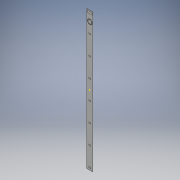
# Autodesk Inventor part: Pieza1
Saved by Autodesk Inventor 2018 (Build 220112000, 112)
## iProperties
Created: 2018-02-27
Part Number: Pieza1
Material: Genérico
Document SubType Name: Modeling
Designer: ivanb
Density: 1 g/cm^3
Appearance: Valor por defecto
Author: ivanb
Autodesk Inventor part; units mm, degrees
ref_plane "YZ Plane" through (0, 0, 0) normal (1, 0, 0) x (0, 1, 0)
ref_plane "XZ Plane" through (0, 0, 0) normal (0, 1, 0) x (-1, 0, 0)
ref_plane "XY Plane" through (0, 0, 0) normal (0, 0, 1) x (1, 0, 0)
sketch "Boceto1" plane through (0, 0, 0) normal (0, 1, 0) x (-1, 0, 0)
  line L0 (-6.5, -143.75) -> (6.5, -143.75)
  line L1 (6.5, -143.75) -> (6.5, 143.75)
  line L2 (6.5, 143.75) -> (-6.5, 143.75)
  line L3 (-6.5, 143.75) -> (-6.5, -143.75)
  line L4 (0, 0) -> (-31.3915, 0)
  line L5 (0, 0) -> (0, -12.323)
  dimension "d0" = 13
  dimension "d1" = 287.5
  constraints: 12 end point, 2 horizontal, 2 parallel, 1 perpendicular, 1 vertical, 2 other
  measures "d0" distance of L2.end L1.end
  measures "d1" distance of L1.end L0.end
extrude "Extrusión1" add sketch "Boceto1" along normal blind 0.16
sketch "Boceto2" plane through (0, 0.16, 0) normal (0, 1, 0) x (1, 0, 0)
  point P0 (0, 0)
sketch "Boceto3" plane through (0, 0.16, 0) normal (0, 1, 0) x (1, 0, 0)
  line L0 (6.5, 143.75) -> (-6.5, 143.75) projected
  line L1 (0, 143.75) -> (0, 97.75)
  line L2 (-2.25, 97.75) -> (2.25, 97.75)
  line L3 (2.25, 97.75) -> (2.25, 100.1)
  line L4 (2.25, 100.1) -> (-2.25, 100.1)
  line L5 (-2.25, 100.1) -> (-2.25, 97.75)
  line L6 (2.25, 57.75) -> (-2.25, 57.75)
  line L7 (-2.25, 57.75) -> (-2.25, 60.1)
  line L8 (-2.25, 60.1) -> (2.25, 60.1)
  line L9 (2.25, 60.1) -> (2.25, 57.75)
  line L10 (2.25, 57.75) -> (-2.25, 60.1) construction
  line L11 (-2.25, 57.75) -> (2.25, 60.1) construction
  line L12 (0, 38.925) -> (-3.2759, 38.925)
  line L13 (0, 78.925) -> (-4.0754, 78.925)
  line L14 (2.25, 20.1) -> (-2.25, 20.1)
  line L15 (-2.25, 20.1) -> (-2.25, 17.75)
  line L16 (-2.25, 17.75) -> (2.25, 17.75)
  line L17 (2.25, 17.75) -> (2.25, 20.1)
  line L18 (2.25, 20.1) -> (-2.25, 17.75) construction
  line L19 (-2.25, 20.1) -> (2.25, 17.75) construction
  line L20 (0, -1.075) -> (-4.0754, -1.075)
  line L21 (0, -41.075) -> (-3.2759, -41.075)
  line L22 (-2.25, -19.9) -> (2.25, -19.9)
  line L23 (2.25, -22.25) -> (-2.25, -22.25)
  line L24 (-2.25, -22.25) -> (-2.25, -19.9)
  line L25 (2.25, -19.9) -> (2.25, -22.25)
  line L26 (-2.25, -22.25) -> (2.25, -19.9) construction
  line L27 (2.25, -22.25) -> (-2.25, -19.9) construction
  line L28 (0, -81.075) -> (-4.0754, -81.075)
  line L29 (2.25, -59.9) -> (-2.25, -59.9)
  line L30 (-2.25, -62.25) -> (2.25, -62.25)
  line L31 (2.25, -62.25) -> (2.25, -59.9)
  line L32 (-2.25, -59.9) -> (2.25, -62.25) construction
  line L33 (2.25, -59.9) -> (-2.25, -62.25) construction
  line L34 (-2.25, -59.9) -> (-2.25, -62.25)
  line L35 (0, -121.075) -> (-3.2759, -121.075)
  line L36 (-2.25, -99.9) -> (2.25, -99.9)
  line L37 (2.25, -102.25) -> (-2.25, -102.25)
  line L38 (2.25, -99.9) -> (2.25, -102.25)
  line L39 (-2.25, -102.25) -> (2.25, -99.9) construction
  line L40 (2.25, -102.25) -> (-2.25, -99.9) construction
  line L41 (-2.25, -102.25) -> (-2.25, -99.9)
  line L42 (0, 118.925) -> (-3.2759, 118.925)
  line L43 (-2.25, 140.1) -> (2.25, 140.1)
  line L44 (2.25, 140.1) -> (2.25, 137.75)
  line L45 (2.25, 137.75) -> (-2.25, 137.75)
  line L46 (-2.25, 137.75) -> (-2.25, 140.1)
  point P0 (0, 0)
  point P1 (0, 98.925)
  point P2 (0, 58.925)
  point P3 (0, 18.925)
  point P4 (0, -21.075)
  point P5 (0, -82.15)
  point P6 (0, -61.075)
  point P7 (0, -101.075)
  point P8 (0, 140.1)
  point P9 (0, 138.925)
  dimension "d4" = 46
  dimension "d5" = 4.5
  dimension "d6" = 2.35
  dimension "d7" = 40
  dimension "d8" = 4.5
  dimension "d9" = 2.35
  dimension "d10" = 20
  dimension "d11" = 20
  constraints: 92 end point, 37 symmetric about line, 11 midpoint, 4 horizontal, 4 parallel, 2 perpendicular, 1 point on line, 1 vertical, 1 other
  measures "d4" distance of L1.start L1.end
  measures "d5" distance of L4.end L3.end
  measures "d6" distance of L3.end L2.end
  measures "d7" distance of point (0, 98.925) point (0, 58.925)
  measures "d8" distance of L6.start L6.end
  measures "d9" distance of L6.end L7.end
  measures "d10" distance from line of L12 point (0, 58.925)
  measures "d11" distance from line of L13 point (0, 98.925)
extrude "Extrusión2" add sketch "Boceto3" along normal blind 1
sketch "Boceto4" plane through (0, 0.16, 0) normal (0, 1, 0) x (1, 0, 0)
  line L0 (-6.5, -143.75) -> (6.5, -143.75) projected
  line L1 (-3.5, -126.25) -> (3.5, -126.25)
  line L2 (3.5, -126.25) -> (3.5, -119.25)
  line L3 (3.5, -119.25) -> (-3.5, -119.25)
  line L4 (-3.5, -119.25) -> (-3.5, -126.25)
  line L5 (-3.5, -126.25) -> (3.5, -119.25) construction
  line L6 (3.5, -126.25) -> (-3.5, -119.25) construction
  point P0 (0, 0)
  point P1 (0, -122.75)
  dimension "d14" = 21
  dimension "d15" = 7
  dimension "d16" = 7
  constraints: 12 end point, 2 midpoint, 2 parallel, 1 horizontal, 1 perpendicular
  measures "d14" distance from line of point (0, -122.75) L0
  measures "d15" distance of L3.end L2.end
  measures "d16" distance of L2.end L1.end
extrude "Extrusión3" add sketch "Boceto4" along normal blind 1
sketch "Boceto5" plane through (0, 0.16, 0) normal (0, 1, 0) x (1, 0, 0)
  line L0 (3.5, -119.25) -> (-3.5, -119.25) projected
  line L1 (-2.7, -119.25) -> (-2.2, -119.25)
  line L2 (-2.2, -119.25) -> (-2.2, -117.9762)
  line L3 (-2.2, -117.9762) -> (-2.7, -117.9762)
  line L4 (-2.7, -117.9762) -> (-2.7, -119.25)
  line L5 (-2, -119.25) -> (-1.5, -119.25)
  line L6 (-1.5, -119.25) -> (-1.5, -117.9762)
  line L7 (-1.5, -117.9762) -> (-2, -117.9762)
  line L8 (-2, -117.9762) -> (-2, -119.25)
  line L9 (-1.3, -119.25) -> (-0.8, -119.25)
  line L10 (-0.8, -119.25) -> (-0.8, -117.9762)
  line L11 (-0.8, -117.9762) -> (-1.3, -117.9762)
  line L12 (-1.3, -117.9762) -> (-1.3, -119.25)
  line L13 (-0.6, -119.25) -> (-0.1, -119.25)
  line L14 (-0.1, -119.25) -> (-0.1, -117.9762)
  line L15 (-0.1, -117.9762) -> (-0.6, -117.9762)
  line L16 (-0.6, -117.9762) -> (-0.6, -119.25)
  line L17 (0.1, -119.25) -> (0.6, -119.25)
  line L18 (0.6, -119.25) -> (0.6, -117.9762)
  line L19 (0.6, -117.9762) -> (0.1, -117.9762)
  line L20 (0.1, -117.9762) -> (0.1, -119.25)
  line L21 (0.8, -119.25) -> (1.3, -119.25)
  line L22 (1.3, -119.25) -> (1.3, -117.9762)
  line L23 (1.3, -117.9762) -> (0.8, -117.9762)
  line L24 (0.8, -117.9762) -> (0.8, -119.25)
  line L25 (1.5, -119.25) -> (2, -119.25)
  line L26 (2, -119.25) -> (2, -117.9762)
  line L27 (2, -117.9762) -> (1.5, -117.9762)
  line L28 (1.5, -117.9762) -> (1.5, -119.25)
  line L29 (2.2, -119.25) -> (2.7, -119.25)
  line L30 (2.7, -119.25) -> (2.7, -117.9762)
  line L31 (2.7, -117.9762) -> (2.2, -117.9762)
  line L32 (2.2, -117.9762) -> (2.2, -119.25)
  line L33 (2.25, -102.25) -> (-2.25, -102.25) projected
  line L34 (0, -102.25) -> (0, -103.6026)
  line L35 (-3.5, -119.25) -> (-3.5, -119.452)
  line L36 (-3.5, -126.25) -> (-3.5, -119.25) projected
  line L37 (-3.5, -119.25) -> (3.5, -119.25) projected
  line L38 (-3.5, -119.25) -> (-3.2852, -119.25)
  line L39 (-3.5, -119.25) -> (-3.5, -126.25) projected
  line L40 (-3.5, -122.75) -> (-4.815, -122.75)
  line L41 (-2.7, -126.25) -> (-2.2, -126.25)
  line L42 (-2.2, -126.25) -> (-2.2, -127.5238)
  line L43 (-2.2, -127.5238) -> (-2.7, -127.5238)
  line L44 (-2.7, -127.5238) -> (-2.7, -126.25)
  line L45 (-2, -126.25) -> (-1.5, -126.25)
  line L46 (-1.5, -126.25) -> (-1.5, -127.5238)
  line L47 (-1.5, -127.5238) -> (-2, -127.5238)
  line L48 (-2, -127.5238) -> (-2, -126.25)
  line L49 (-1.3, -126.25) -> (-0.8, -126.25)
  line L50 (-0.8, -126.25) -> (-0.8, -127.5238)
  line L51 (-0.8, -127.5238) -> (-1.3, -127.5238)
  line L52 (-1.3, -127.5238) -> (-1.3, -126.25)
  line L53 (-0.6, -126.25) -> (-0.1, -126.25)
  line L54 (-0.1, -126.25) -> (-0.1, -127.5238)
  line L55 (-0.1, -127.5238) -> (-0.6, -127.5238)
  line L56 (-0.6, -127.5238) -> (-0.6, -126.25)
  line L57 (0.1, -126.25) -> (0.6, -126.25)
  line L58 (0.6, -126.25) -> (0.6, -127.5238)
  line L59 (0.6, -127.5238) -> (0.1, -127.5238)
  line L60 (0.1, -127.5238) -> (0.1, -126.25)
  line L61 (0.8, -126.25) -> (1.3, -126.25)
  line L62 (1.3, -126.25) -> (1.3, -127.5238)
  line L63 (1.3, -127.5238) -> (0.8, -127.5238)
  line L64 (0.8, -127.5238) -> (0.8, -126.25)
  line L65 (1.5, -126.25) -> (2, -126.25)
  line L66 (2, -126.25) -> (2, -127.5238)
  line L67 (2, -127.5238) -> (1.5, -127.5238)
  line L68 (1.5, -127.5238) -> (1.5, -126.25)
  line L69 (2.2, -126.25) -> (2.7, -126.25)
  line L70 (2.7, -126.25) -> (2.7, -127.5238)
  line L71 (2.7, -127.5238) -> (2.2, -127.5238)
  line L72 (2.2, -127.5238) -> (2.2, -126.25)
  line L73 (-4.6545, -125.45) -> (-3.5, -125.45)
  line L74 (-3.5, -125.45) -> (-3.5, -124.95)
  line L75 (-3.5, -124.95) -> (-4.6545, -124.95)
  line L76 (-4.6545, -124.95) -> (-4.6545, -125.45)
  line L77 (-4.6545, -124.75) -> (-3.5, -124.75)
  line L78 (-3.5, -124.75) -> (-3.5, -124.25)
  line L79 (-3.5, -124.25) -> (-4.6545, -124.25)
  line L80 (-4.6545, -124.25) -> (-4.6545, -124.75)
  line L81 (-4.6545, -124.05) -> (-3.5, -124.05)
  line L82 (-3.5, -124.05) -> (-3.5, -123.55)
  line L83 (-3.5, -123.55) -> (-4.6545, -123.55)
  line L84 (-4.6545, -123.55) -> (-4.6545, -124.05)
  line L85 (-4.6545, -123.35) -> (-3.5, -123.35)
  line L86 (-3.5, -123.35) -> (-3.5, -122.85)
  line L87 (-3.5, -122.85) -> (-4.6545, -122.85)
  line L88 (-4.6545, -122.85) -> (-4.6545, -123.35)
  line L89 (-4.6545, -122.65) -> (-3.5, -122.65)
  line L90 (-3.5, -122.65) -> (-3.5, -122.15)
  line L91 (-3.5, -122.15) -> (-4.6545, -122.15)
  line L92 (-4.6545, -122.15) -> (-4.6545, -122.65)
  line L93 (-4.6545, -121.95) -> (-3.5, -121.95)
  line L94 (-3.5, -121.95) -> (-3.5, -121.45)
  line L95 (-3.5, -121.45) -> (-4.6545, -121.45)
  line L96 (-4.6545, -121.45) -> (-4.6545, -121.95)
  line L97 (-4.6545, -121.25) -> (-3.5, -121.25)
  line L98 (-3.5, -121.25) -> (-3.5, -120.75)
  line L99 (-3.5, -120.75) -> (-4.6545, -120.75)
  line L100 (-4.6545, -120.75) -> (-4.6545, -121.25)
  line L101 (-4.6545, -120.55) -> (-3.5, -120.55)
  line L102 (-3.5, -120.55) -> (-3.5, -120.05)
  line L103 (-3.5, -120.05) -> (-4.6545, -120.05)
  line L104 (-4.6545, -120.05) -> (-4.6545, -120.55)
  line L105 (3.5, -119.25) -> (3.5, -126.25) projected
  line L106 (3.5, -122.75) -> (2.5278, -122.75)
  line L107 (0, -119.25) -> (0, -116.7727)
  line L108 (3.5, -122.75) -> (4.815, -122.75)
  line L109 (4.6545, -125.45) -> (3.5, -125.45)
  line L110 (3.5, -125.45) -> (3.5, -124.95)
  line L111 (3.5, -124.95) -> (4.6545, -124.95)
  line L112 (4.6545, -124.95) -> (4.6545, -125.45)
  line L113 (3.5, -124.25) -> (4.6545, -124.25)
  line L114 (3.5, -124.75) -> (3.5, -124.25)
  line L115 (4.6545, -124.75) -> (3.5, -124.75)
  line L116 (4.6545, -124.25) -> (4.6545, -124.75)
  line L117 (3.5, -123.55) -> (4.6545, -123.55)
  line L118 (3.5, -124.05) -> (3.5, -123.55)
  line L119 (4.6545, -124.05) -> (3.5, -124.05)
  line L120 (4.6545, -123.55) -> (4.6545, -124.05)
  line L121 (3.5, -122.85) -> (4.6545, -122.85)
  line L122 (3.5, -123.35) -> (3.5, -122.85)
  line L123 (4.6545, -123.35) -> (3.5, -123.35)
  line L124 (4.6545, -122.85) -> (4.6545, -123.35)
  line L125 (3.5, -122.15) -> (4.6545, -122.15)
  line L126 (3.5, -122.65) -> (3.5, -122.15)
  line L127 (4.6545, -122.65) -> (3.5, -122.65)
  line L128 (4.6545, -122.15) -> (4.6545, -122.65)
  line L129 (3.5, -121.45) -> (4.6545, -121.45)
  line L130 (3.5, -121.95) -> (3.5, -121.45)
  line L131 (4.6545, -121.95) -> (3.5, -121.95)
  line L132 (4.6545, -121.45) -> (4.6545, -121.95)
  line L133 (3.5, -120.75) -> (4.6545, -120.75)
  line L134 (3.5, -121.25) -> (3.5, -120.75)
  line L135 (4.6545, -121.25) -> (3.5, -121.25)
  line L136 (4.6545, -120.75) -> (4.6545, -121.25)
  line L137 (3.5, -120.05) -> (4.6545, -120.05)
  line L138 (3.5, -120.55) -> (3.5, -120.05)
  line L139 (4.6545, -120.55) -> (3.5, -120.55)
  line L140 (4.6545, -120.05) -> (4.6545, -120.55)
  point P0 (0, 0)
  dimension "d19" = 0.2
  dimension "d20" = 0.2
  dimension "d21" = 0.2
  dimension "d22" = 0.2
  dimension "d23" = 0.2
  dimension "d24" = 0.2
  dimension "d25" = 0.2
  dimension "d26" = 0.5
  dimension "d27" = 0.5
  dimension "d28" = 0.5
  dimension "d29" = 0.5
  dimension "d30" = 0.5
  dimension "d31" = 0.5
  dimension "d32" = 0.5
  dimension "d33" = 0.5
  dimension "d36" = 1.2738
  dimension "d37" = 0.5
  dimension "d38" = 0.5
  dimension "d39" = 0.5
  dimension "d40" = 0.5
  dimension "d41" = 0.5
  dimension "d42" = 0.5
  dimension "d43" = 0.5
  dimension "d44" = 0.5
  dimension "d45" = 0.2
  dimension "d46" = 0.2
  dimension "d47" = 0.2
  dimension "d48" = 0.2
  dimension "d49" = 0.2
  dimension "d50" = 0.2
  dimension "d51" = 0.2
  constraints: 270 end point, 66 symmetric about line, 32 parallel, 18 horizontal, 16 perpendicular, 3 midpoint, 3 point on line, 2 vertical, 5 other
  measures "d19" distance between parallel lines of L8 L2
  measures "d20" distance between parallel lines of L12 L6
  measures "d21" distance between parallel lines of L16 L10
  measures "d22" distance between parallel lines of L14 L20
  measures "d23" distance between parallel lines of L18 L24
  measures "d24" distance between parallel lines of L22 L28
  measures "d25" distance between parallel lines of L26 L32
  measures "d26" distance of L2.end L3.end
  measures "d27" distance of L6.end L7.end
  measures "d28" distance of L10.end L11.end
  measures "d29" distance of L14.end L15.end
  measures "d30" distance of L18.end L19.end
  measures "d31" distance of L22.end L23.end
  measures "d32" distance of L26.end L27.end
  measures "d33" distance of L30.end L31.end
  measures "d36" distance of L44.start L41.start
  measures "d37" distance of L74.end L73.end
  measures "d38" distance of L79.start L78.start
  measures "d39" distance of L83.start L82.start
  measures "d40" distance of L87.start L86.start
  measures "d41" distance of L91.start L90.start
  measures "d42" distance of L95.start L94.start
  measures "d43" distance of L99.start L98.start
  measures "d44" distance of L103.start L102.start
  measures "d45" distance between parallel lines of L77 L75
  measures "d46" distance between parallel lines of L81 L79
  measures "d47" distance between parallel lines of L85 L83
  measures "d48" distance between parallel lines of L89 L87
  measures "d49" distance between parallel lines of L93 L91
  measures "d50" distance between parallel lines of L97 L95
  measures "d51" distance between parallel lines of L101 L99
extrude "Extrusión4" add sketch "Boceto5" along normal blind 0.5
sketch "Boceto6" plane through (0, 0.16, 0) normal (0, 1, 0) x (1, 0, 0)
  line L0 (-4.6, -141.25) -> (4.6, -141.25)
  line L1 (4.6, -141.25) -> (4.6, -136.95)
  line L2 (4.6, -136.95) -> (-4.6, -136.95)
  line L3 (-4.6, -136.95) -> (-4.6, -141.25)
  line L4 (-6.5, -143.75) -> (6.5, -143.75) projected
  line L5 (0, -143.75) -> (0, -142.0268)
  line L6 (-5.4569, -141.25) -> (5.4569, -141.25)
  line L7 (5.4569, -141.25) -> (5.4569, -140.75)
  line L8 (5.4569, -140.75) -> (-5.4569, -140.75)
  line L9 (-5.4569, -140.75) -> (-5.4569, -141.25)
  point P0 (0, 0)
  dimension "d52" = 9.2
  dimension "d53" = 4.3
  dimension "d54" = 2.5
  dimension "d55" = 0.5
  constraints: 18 end point, 4 parallel, 2 horizontal, 2 perpendicular, 1 midpoint, 1 vertical, 2 other
  measures "d52" distance of L2.end L1.end
  measures "d53" distance of L1.end L0.end
  measures "d54" distance between parallel lines of L4 L0
  measures "d55" distance of L7.end L6.end
extrude "Extrusión5" add sketch "Boceto6" along normal blind 0.5
